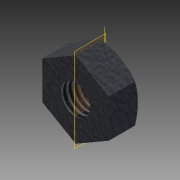
# Autodesk Inventor part: M8_driving_nut
Saved by Autodesk Inventor 2015 (Build 190159000, 159)
## iProperties
Created: 2013-12-24
Part Number: M8_driving_nut
Material: Generic
Document SubType Name: Modeling
Designer: aoki
Density: 1 g/cm^3
Appearance: Iron - Cast
Author: aoki
Autodesk Inventor part; units mm, degrees
ref_plane "XZ Plane" through (0, 0, 0) normal (0, 1, 0) x (-1, 0, 0)
ref_plane "XY Plane" through (0, 0, 0) normal (0, 0, 1) x (1, 0, 0)
sketch "Sketch1" plane through (0, 0, 0) normal (0, 1, 0) x (-1, 0, 0)
  line L0 (7.5, -4.3301) -> (0, -8.6603)
  line L1 (0, -8.6603) -> (-7.5, -4.3301)
  line L2 (-7.5, -4.3301) -> (-7.5, 4.3301)
  line L3 (-7.5, 4.3301) -> (0, 8.6603)
  line L4 (0, 8.6603) -> (7.5, 4.3301)
  line L5 (7.5, 4.3301) -> (7.5, -4.3301)
  point P0 (0, 0)
  point P1 (0, 0)
  dimension "d0" = 15
  constraints: 12 end point, 1 coincident, 1 vertical, 13 other
  measures "d0" distance between parallel lines of L5 L2
extrude "Extrusion1" add sketch "Sketch1" against normal blind 6.5
sketch "Sketch2" plane through (0, 0, 0) normal (1, 0, 0) x (0, 1, 0)
  point P0 (0, 0)
ref_plane "Work Plane2" through (0, 0, 0) normal (1, 0, 0) x (0, 0, 1)
sketch "Sketch6" plane through (0, 0, 0) normal (1, 0, 0) x (0, 1, 0)
  line L0 (0, 8.6603) -> (0, 4.3301) projected
  line L1 (0, 4.3301) -> (-6.5, 4.3301) projected
  line L2 (-6.5, 8.6603) -> (-6.5, 4.3301) projected
  line L3 (0, 8.6603) -> (-6.5, 8.6603) projected
  line L4 (0, 8.6603) -> (0, 7.6603)
  line L5 (-0.5774, 8.6603) -> (0, 8.6603)
  line L6 (-0.5774, 8.6603) -> (0, 7.6603)
  line L7 (-0.3756, 0) -> (-10.093, 0)
  point P0 (0, 0)
  dimension "d6" = 1
  dimension "d7" = 30
  constraints: 8 end point, 2 point on line, 1 collinear, 1 parallel, 1 perpendicular
  measures "d6" distance of L4.end L0.start
  measures "d7" angle of L0 L6
revolve "Revolution1" cut sketch "Sketch6" angle 360 about axis through (0, -0.3756, 0) along (0, -1, 0) contours L0 L6 L3
sketch "Sketch7" plane through (0, 0, 0) normal (0, 1, 0) x (1, 0, 0)
  arc A0 (-5.0999, 5.7158) -> (-7.5, 1.5587) centre (0, 0) ccw projected
  constraints: 1 coincident
hole "Hole1" at (0, 0, 0) direction (0, -1, 0) diameter 6.647 end through all thread size "M8x1.25" class "6H" standard "ANSI Metric M Profile"
body "Solid1"
